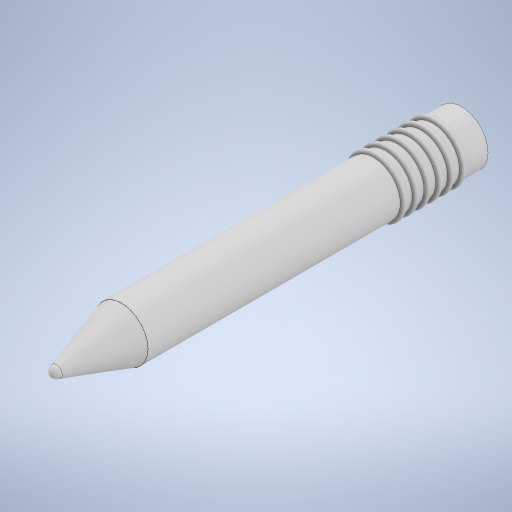
# Autodesk Inventor part: srb_body
Saved by Autodesk Inventor 2024 (Build 280153000, 153)
## iProperties
Created: 2023-06-07
Part Number: srb_body
Material: Generic
Document SubType Name: Modeling
Designer: tamiz
Density: 1 g/cm^3
Appearance: Default
Author: tamiz
Autodesk Inventor part; units mm, degrees
ref_plane "YZ Plane" through (0, 0, 0) normal (1, 0, 0) x (0, 1, 0)
ref_plane "XZ Plane" through (0, 0, 0) normal (0, 1, 0) x (-1, 0, 0)
ref_plane "XY Plane" through (0, 0, 0) normal (0, 0, 1) x (1, 0, 0)
sketch "Sketch2" plane through (0, 0, 0) normal (0, 0, 1) x (1, 0, 0)
  circle A0 centre (0, 0) radius 2743.2
  dimension "d0" = 5486.4
  constraints: 1 centre point, 1 coincident
  measures "d0" diameter of A0
extrude "Extrusion1" add sketch "Sketch2" along normal mid plane 35052
ref_plane "Work Plane1" through (0, 0, 24231.6) normal (0, 0, 1) x (1, 0, 0)
sketch "Sketch3" plane through (0, 0, 24231.6) normal (0, 0, 1) x (1, 0, 0)
  circle A0 centre (0, 0) radius 609.6
  dimension "d4" = 1219.2
  constraints: 1 centre point, 1 coincident
  measures "d4" diameter of A0
extrude "Extrusion2" add sketch "Sketch3" against normal blind 6705.6 draft 17.5
sketch "Sketch4" plane through (0, 0, 24231.6) normal (0, 0, 1) x (1, 0, 0)
  arc A0 (609.6, 0) -> (-609.6, 0) centre (0, 0) ccw
  line L0 (-609.6, 0) -> (609.6, 0)
  constraints: 2 end point, 2 point on circle, 1 centre point, 1 coincident, 1 horizontal
revolve "Revolution1" add sketch "Sketch4" angle 180 about axis through (-609.6, 0, 24231.6) along (1, 0, 0)
sketch "Sketch5" plane through (0, 0, 0) normal (1, 0, 0) x (0, 1, 0)
  arc A0 (2743.2, -15191.1046) -> (2743.2, -14581.5046) centre (2743.2, -14886.3046) ccw
  arc A1 (2743.2, -13971.9046) -> (2743.2, -13362.3046) centre (2743.2, -13667.1046) ccw
  arc A2 (2743.2, -12752.7046) -> (2743.2, -12143.1046) centre (2743.2, -12447.9046) ccw
  arc A3 (2743.2, -11533.5046) -> (2743.2, -10923.9046) centre (2743.2, -11228.7046) ccw
  arc A4 (2743.2, -10314.3046) -> (2743.2, -9704.7046) centre (2743.2, -10009.5046) ccw
  arc A5 (2743.2, -9095.1046) -> (2743.2, -8485.5046) centre (2743.2, -8790.3046) ccw
  line L0 (0, -20453.2822) -> (0, 20694.7178) construction
  line L1 (2743.2, -8485.5046) -> (2743.2, -9095.1046)
  line L2 (2743.2, -17526) -> (2743.2, 17526) projected
  line L3 (2743.2, -9704.7046) -> (2743.2, -10314.3046)
  line L4 (2743.2, -17526) -> (2743.2, 17526) projected
  line L5 (2743.2, -10923.9046) -> (2743.2, -11533.5046)
  line L6 (2743.2, -17526) -> (2743.2, 17526) projected
  line L7 (2743.2, -12143.1046) -> (2743.2, -12752.7046)
  line L8 (2743.2, -13362.3046) -> (2743.2, -13971.9046)
  line L9 (2743.2, -17526) -> (2743.2, 17526) projected
  line L10 (2743.2, -14581.5046) -> (2743.2, -15191.1046)
  line L11 (2743.2, -17526) -> (2743.2, 17526) projected
  point P0 (0, 0)
  dimension "d8" = 609.6
  dimension "d14" = 609.6
  dimension "d15" = 609.6
  dimension "d16" = 609.6
  dimension "d17" = 609.6
  dimension "d18" = 609.6
  dimension "d24" = 41148
  constraints: 14 end point, 12 point on circle, 6 centre point, 4 collinear, 3 vertical, 2 other
  measures "d8" diameter of A0
  measures "d14" diameter of A1
  measures "d15" diameter of A2
  measures "d16" diameter of A3
  measures "d17" diameter of A4
  measures "d18" diameter of A5
  measures "d24" distance of L0.start L0.end
sketch "Sketch6" plane through (0, 0, 24231.6) normal (0, 0, 1) x (1, 0, 0)
  circle A0 centre (0, 0) radius 114.9647
  constraints: 1 centre point, 1 coincident
extrude "Extrusion3" cut sketch "Sketch6" against normal blind 6705.6 draft 18
sketch "Sketch7" plane through (0, 0, 17526) normal (0, 0, 1) x (1, 0, 0)
  point P0 (0, 0)
sketch "Sketch8" plane through (0, 0, -17526) normal (0, 0, -1) x (-1, 0, 0)
  circle A0 centre (0, 0) radius 2743.2
  circle A1 centre (0, 0) radius 2286
  dimension "d21" = 457.2
  constraints: 2 centre point, 1 coincident
  measures "d21" radial gap between concentric circles of A0 A1
extrude "Extrusion4" cut sketch "Sketch8" against normal blind 35661.6 contours A1
revolve "Revolution2" add sketch "Sketch5" angle 360 about axis through (0, 0, -20453.2822) along (0, 0, 1)
body "Solid1"
